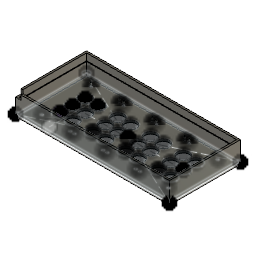
ClockClock24_4Screens (Autodesk Fusion 360 design; units mm, degrees)
Autodesk Fusion 360 part; units mm, degrees
sketch "Sketch1" plane through (0, 0, 0) normal (0, 0, 1) x (1, 0, 0)
  circle A0 centre (0, 0) radius 9.15
  circle A1 centre (19.4, 0) radius 9.15
  circle A2 centre (0, 19.4) radius 9.15
  circle A3 centre (19.4, 19.4) radius 9.15
  circle A4 centre (0, 38.8) radius 9.15
  circle A5 centre (19.4, 38.8) radius 9.15
  circle A6 centre (50.5, 19.4) radius 9.15
  circle A7 centre (69.9, 19.4) radius 9.15
  circle A8 centre (69.9, 0) radius 9.15
  circle A9 centre (50.5, 38.8) radius 9.15
  circle A10 centre (50.5, 0) radius 9.15
  circle A11 centre (69.9, 38.8) radius 9.15
  circle A12 centre (101, 19.4) radius 9.15
  circle A13 centre (120.4, 19.4) radius 9.15
  circle A14 centre (120.4, 0) radius 9.15
  circle A15 centre (101, 38.8) radius 9.15
  circle A16 centre (101, 0) radius 9.15
  circle A17 centre (120.4, 38.8) radius 9.15
  circle A18 centre (151.5, 19.4) radius 9.15
  circle A19 centre (170.9, 19.4) radius 9.15
  circle A20 centre (170.9, 0) radius 9.15
  circle A21 centre (151.5, 38.8) radius 9.15
  circle A22 centre (151.5, 0) radius 9.15
  circle A23 centre (170.9, 38.8) radius 9.15
  line L0 (0, 19.4) -> (170.9, 19.4) construction
  line L1 (204.4, 74.3) -> (-33.5, 74.3)
  line L2 (-33.5, 74.3) -> (-33.5, -35.5)
  line L3 (-33.5, -35.5) -> (204.4, -35.5)
  line L4 (204.4, -35.5) -> (204.4, 74.3)
  line L5 (204.4, 74.3) -> (-33.5, -35.5) construction
  line L6 (-33.5, 74.3) -> (204.4, -35.5) construction
  circle A24 centre (-12.4, 60.05) radius 1.5
  circle A25 centre (31.8, 60.05) radius 1.5
  circle A26 centre (-12.4, -15.94) radius 1.5
  circle A27 centre (31.8, -15.94) radius 1.5
  line L7 (0, 38.8) -> (19.4, 38.8) construction
  line L8 (9.7, 38.8) -> (9.7, -26) construction
  circle A28 centre (38.1, 60.05) radius 1.5
  circle A29 centre (82.3, 60.05) radius 1.5
  circle A30 centre (82.3, -15.94) radius 1.5
  circle A31 centre (38.1, -15.94) radius 1.5
  circle A32 centre (88.6, 60.05) radius 1.5
  circle A33 centre (132.8, 60.05) radius 1.5
  circle A34 centre (132.8, -15.94) radius 1.5
  circle A35 centre (88.6, -15.94) radius 1.5
  circle A36 centre (139.1, 60.05) radius 1.5
  circle A37 centre (183.3, 60.05) radius 1.5
  circle A38 centre (183.3, -15.94) radius 1.5
  circle A39 centre (139.1, -15.94) radius 1.5
  arc A40 (-28.5, 74.3) -> (-33.5, 69.3) centre (-33.5, 74.3) ccw
  arc A41 (-33.5, -30.5) -> (-28.5, -35.5) centre (-33.5, -35.5) ccw
  arc A42 (199.4, -35.5) -> (204.4, -30.5) centre (204.4, -35.5) ccw
  arc A43 (204.4, 69.3) -> (199.4, 74.3) centre (204.4, 74.3) ccw
  line L9 (-33.5, 69.8) -> (-33.6, 69.8)
  line L10 (-33.6, 69.8) -> (-33.6, 74.4)
  line L11 (-33.6, 74.4) -> (-29, 74.4)
  line L12 (-29, 74.4) -> (-29, 74.3)
  line L13 (199.9, 74.3) -> (199.9, 74.4)
  line L14 (199.9, 74.4) -> (204.5, 74.4)
  line L15 (204.5, 74.4) -> (204.5, 69.8)
  line L16 (204.5, 69.8) -> (204.4, 69.8)
  line L17 (199.9, -35.5) -> (199.9, -35.6)
  line L18 (199.9, -35.6) -> (204.5, -35.6)
  line L19 (204.5, -35.6) -> (204.5, -31)
  line L20 (204.5, -31) -> (204.4, -31)
  line L21 (-29, -35.5) -> (-29, -35.6)
  line L22 (-29, -35.6) -> (-33.6, -35.6)
  line L23 (-33.6, -35.6) -> (-33.6, -31)
  line L24 (-33.6, -31) -> (-33.5, -31)
  line L25 (200.4, 70.3) -> (-29.5, 70.3)
  line L26 (-29.5, 70.3) -> (-29.5, -31.5)
  line L27 (-29.5, -31.5) -> (200.4, -31.5)
  line L28 (200.4, -31.5) -> (200.4, 70.3)
  point P0 (50.5, 0)
  point P1 (101, 0)
  point P2 (151.5, 0)
  point P3 (85.45, 19.4)
  point P4 (85.45, 19.4)
  dimension "d1" = 18.3
  dimension "d4" = 19.4
  dimension "d5" = 38.8
  dimension "d13" = 151.5
  dimension "d14" = 0
  dimension "d22" = 237.9
  dimension "d23" = 109.8
  dimension "d25" = 3
  dimension "d28" = 44.2
  dimension "d29" = -75.99
  dimension "d31" = 22.1
  dimension "d32" = 22.1
  dimension "d33" = 21.25
  dimension "d37" = 151.5
  dimension "d38" = 0
  dimension "d48" = 10
  dimension "d49" = 10
  dimension "d50" = 10
  dimension "d51" = 10
  dimension "d55" = 0.1
  dimension "d56" = 0.1
  dimension "d57" = 0.1
  dimension "d58" = 0.1
  dimension "d59" = 0.1
  dimension "d60" = 0.1
  dimension "d61" = 0.1
  dimension "d62" = 0.1
  dimension "d63" = 4.5
  dimension "d64" = 4.5
  dimension "d65" = 4.5
  dimension "d66" = 4.5
  dimension "d67" = 4.5
  dimension "d68" = 4.5
  dimension "d69" = 4.5
  dimension "d70" = 4.5
  dimension "d76" = -4
  constraint coincident A0.centre origin
  constraint coincident A2.centre L0.start
  constraint coincident A19.centre L0.end
  constraint midpoint L0 P4
  constraint horizontal L1
  constraint perpendicular L1 L2
  constraint parallel L1 L3
  constraint parallel L2 L4
  constraint coincident L5 P4
  constraint coincident L6 P4
  constraint coincident P4 P3
  constraint coincident A4.centre L7.start
  constraint coincident A5.centre L7.end
  constraint midpoint L7 L8.start
  constraint perpendicular L7 L8
  constraint coincident L1.end L2.start
  constraint coincident L1.start L4.end
  constraint coincident L3.end L4.start
  constraint coincident L2.end L3.start
  constraint coincident L2 A40.end
  constraint coincident L1 A40.start
  constraint coincident L2 A41.start
  constraint coincident L3 A41.end
  constraint coincident L4 A42.end
  constraint coincident L3 A42.start
  constraint coincident L1 A43.end
  constraint coincident L4 A43.start
  constraint coincident L2 L9.start
  constraint perpendicular L2 L9
  constraint perpendicular L9 L10
  constraint perpendicular L10 L11
  constraint coincident L1 L12.end
  constraint perpendicular L1 L12
  constraint coincident L1 L13.start
  constraint perpendicular L1 L13
  constraint perpendicular L13 L14
  constraint perpendicular L14 L15
  constraint coincident L4 L16.end
  constraint perpendicular L4 L16
  constraint coincident L3 L17.start
  constraint perpendicular L3 L17
  constraint perpendicular L17 L18
  constraint perpendicular L3 L19
  constraint coincident L4 L20.end
  constraint perpendicular L4 L20
  constraint coincident L3 L21.start
  constraint perpendicular L3 L21
  constraint perpendicular L21 L22
  constraint perpendicular L22 L23
  constraint coincident L2 L24.end
  constraint perpendicular L2 L24
  measures "d1" diameter of A0
  measures "d22" distance of L1.start L1.end
  measures "d23" distance of L1.end L2.end
  measures "d25" diameter of A24
  measures "d31" distance of A24.centre L8
  measures "d32" distance of A25.centre L8
  measures "d33" vertical distance of A4.centre A24.centre
  measures "d48" diameter of A40
  measures "d49" diameter of A43
  measures "d50" diameter of A42
  measures "d51" diameter of A41
  measures "d55" distance of L2 L23
  measures "d56" distance of L3 L22
  measures "d57" distance of L1 L11
  measures "d58" distance of L2 L10
  measures "d59" distance of L1 L14
  measures "d60" distance of L4 L15
  measures "d61" distance of L4 L19
  measures "d62" distance of L3 L18
  measures "d63" distance of L1.end L12
  measures "d64" distance of L1.end L9
  measures "d65" distance of L1.start L16
  measures "d66" distance of L1.start L13
  measures "d67" distance of L3.end L20
  measures "d68" distance of L3.end L17
  measures "d69" distance of L2.end L21
  measures "d70" distance of L2.end L24
extrude "Extrude1" add sketch "Sketch1" against normal blind 3 contours L1 L2 L3 L4 | A24 | A25 | A26 | A27 | A28 | A29 | A30 | A31 | A32 | A33 | A34 | A35 | A36 | A37 | A38 | A39 | L25 L26 L27 L28 makes body 1
extrude "Extrude2" add sketch "Sketch1" along normal blind 6 contours A24 | A25 | A26 | A27 | A28 | A29 | A30 | A31 | A32 | A33 | A34 | A35 | A36 | A37 | A38 | A39 bodies 1
chamfer "Chamfer1" distance 0.3 angle 85 16 edges at (-13.7985, -16.4824, 6) (30.4015, -16.4824, 6) (36.7015, -16.4824, 6) (80.9015, -16.4824, 6) (87.2015, -16.4824, 6) (131.4015, -16.4824, 6) (137.7015, -16.4824, 6) (181.9015, -16.4824, 6) (181.9015, 59.5076, 6) (137.7015, 59.5076, 6) (131.4015, 59.5076, 6) (87.2015, 59.5076, 6) (80.9015, 59.5076, 6) (36.7015, 59.5076, 6) (30.4015, 59.5076, 6) (-13.7985, 59.5076, 6) measured on face at (-12.8778, -15.4072, 6) measured on face at (32.1887, -15.4525, 6) measured on face at (37.7279, -15.6744, 6) measured on face at (81.7657, -16.3309, 6) measured on face at (88.0657, -16.3309, 6) measured on face at (132.0681, -16.2801, 6) measured on face at (138.3681, -16.2801, 6) measured on face at (182.5681, -16.2801, 6) measured on face at (183.4113, 59.5625, 6) measured on face at (139.2113, 59.5625, 6) measured on face at (132.9113, 59.5625, 6) measured on face at (88.7113, 59.5625, 6) measured on face at (82.4113, 59.5625, 6) measured on face at (38.8169, 59.9755, 6) measured on face at (32.5003, 59.9026, 6) measured on face at (-13.2158, 59.8331, 6) on bodies 1
extrude "Extrude3" add sketch "Sketch1" along normal blind 30 thin wall 3 on the right open curves L1 L2 L3 L4 bodies 1
sketch "Sketch2" plane through (0, 0, 30) normal (0, 0, 1) x (-1, 0, 0)
  line L0 (-201.4, -71.3) -> (-201.4, 32.5)
  line L1 (-201.4, 32.5) -> (30.5, 32.5)
  line L2 (30.5, 32.5) -> (30.5, -71.3)
  line L3 (30.5, -71.3) -> (-201.4, -71.3)
  line L4 (-204.4, -74.3) -> (33.5, -74.3)
  line L5 (33.5, -74.3) -> (33.5, 35.5)
  line L6 (33.5, 35.5) -> (-204.4, 35.5)
  line L7 (-204.4, 35.5) -> (-204.4, -74.3)
  line L8 (33.5, 35.5) -> (25, 35.5)
  line L9 (25, 35.5) -> (25, 27)
  line L10 (25, 27) -> (33.5, 27)
  line L11 (33.5, 27) -> (33.5, 35.5)
  constraint horizontal L8
  constraint vertical L9
  constraint horizontal L10
  constraint vertical L11
  constraint coincident L5.end L6.start
extrude "Extrude4" cut sketch "Sketch2" against normal blind 7 contours L1 L2 L5 L6 L8 L9 L10 L11 bodies 1
extrude "Extrude5" [suppressed]
extrude "Extrude6" add sketch "Sketch1" along normal blind 0.4 separate body contours L1 L2 L3 L4 | L25 L26 L27 L28 makes body 2
move_face "OffsetFaces1" offset -4 4 faces at (-33.5, 37.7, 0.1333) (125.1, -35.5, 0.2667) (204.4, 1.1, 0.1333) (45.8, 74.3, 0.2667) on bodies 2
move_face "OffsetFaces2" offset -0.2 16 faces at (139.7843, 61.3848, 0.1333) (183.9843, 61.3848, 0.1333) (133.4843, 61.3848, 0.1333) (90.0095, 60.563, 0.1333) (83.7095, 60.563, 0.1333) (39.5095, 60.563, 0.1333) (33.2095, 60.563, 0.1333) (-10.9905, 60.563, 0.1333) (-10.9019, -15.8652, 0.1333) (32.2777, -14.5181, 0.1333) (38.5777, -14.5181, 0.1333) (81.3075, -17.0647, 0.2667) (87.6075, -17.0647, 0.2667) (133.4843, -14.6052, 0.1333) (139.7843, -14.6052, 0.1333) (183.9843, -14.6052, 0.1333) on bodies 2
extrude "Extrude7" add sketch "Sketch1" along normal blind 20 thin wall 1 centred open curves L26 L27 L28 L25 bodies 2
equation "d1 = clock_dia"
equation "d4 = clock_dist_center"
equation "d5 = clock_dist_center * 2"
equation "clock_dia = 18.3 mm"
equation "clock_dist = 1.1 mm"
equation "clock_dist_center = clock_dia + clock_dist"
equation "clock_digit_dist = 12.8 mm"
equation "clock_digit_dist_center = clock_dia + clock_digit_dist + clock_dist_center"
equation "d13 = clock_digit_dist_center * 3"
equation "d15 = -cover_height"
equation "cover_height = 3 mm"
equation "d22 = clock_dia * 13"
equation "d23 = clock_dia * 6"
equation "test = clock_dia * 5 + 2 * clock_dist + 3 * clock_digit_dist"
equation "d33 = clock_dia / 2 + dist_circle_top + 1.5 mm"
equation "dist_circle_top = 10.6 mm"
equation "d37 = 3 * ( 2 * clock_dia + clock_digit_dist + clock_dist )"
equation "d55 = ear_dist"
equation "d56 = ear_dist"
equation "d57 = ear_dist"
equation "d58 = ear_dist"
equation "d59 = ear_dist"
equation "d60 = ear_dist"
equation "d61 = ear_dist"
equation "d62 = ear_dist"
equation "ear_dist = 0.1 mm"
named bodies: "ClockClock24Body", "CloclClocl24Blocker"
